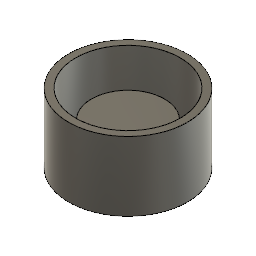
laserCapBottom (Autodesk Fusion 360 design; units mm, degrees)
Autodesk Fusion 360 part; units mm, degrees
sketch "Sketch1" plane through (0, 0, 0) normal (0, 1, 0) x (1, 0, 0)
  circle A0 centre (0, 0) radius 15
  dimension "d1" = 30
  measures "d1" diameter of A0
extrude "Extrude1" add sketch "Sketch1" along normal blind 3.5
ref_plane "WorkPlane1" through (0, 3.5, 0) normal (0, 1, 0) x (1, 0, 0)
sketch "Sketch2" plane through (0, 3.5, 0) normal (0, 1, 0) x (1, 0, 0)
  circle A0 centre (0, 0) radius 9.2075
  dimension "d5" = 18.415
  measures "d5" diameter of A0
extrude "Extrude2" add sketch "Sketch2" along normal blind 7
ref_plane "WorkPlane2" through (0, 3.5, 0) normal (0, 1, 0) x (1, 0, 0)
sketch "Sketch3" plane through (0, 3.5, 0) normal (0, 1, 0) x (1, 0, 0)
  circle A0 centre (0, 0) radius 15
  circle A1 centre (0, 0) radius 13.2
  dimension "d9" = 26.4
  measures "d9" diameter of A1
extrude "Extrude3" add sketch "Sketch3" along normal blind 14
